Autodesk Fusion 360 part; units mm, degrees
(part 3 of 4)
sketch "Sketch4" plane through (0, 0, 0) normal (0, 0, -1) x (1, 0, 0) in component "Gear "
  line L0 (24.6001, -83.7803) -> (24.6516, -83.9556)
  line L1 (24.6516, -83.9556) -> (24.6577, -83.8757)
  line L2 (24.6577, -83.8757) -> (24.6976, -83.9421)
  line L3 (24.6976, -83.9421) -> (24.6684, -83.7391)
  spline S0 degree 5 poles (24.6684, -83.7391) (24.7188, -83.1041) (24.8375, -81.8379) (25.0626, -80.0652) (25.4578, -77.9934) (26.1207, -75.9415) (26.9802, -74.4769) (28.0438, -73.6781) (29.3213, -73.5772) (30.8056, -74.151) (32.4625, -75.3371) (33.9214, -76.7307) (35.082, -78.0047) (35.8789, -78.9461) (36.2729, -79.4266) knots 0.006357 0.006357 0.006357 0.006357 0.006357 0.006357 0.1 0.2 0.3 0.4 0.5 0.6 0.7 0.8 0.9 0.994293 0.994293 0.994293 0.994293 0.994293 0.994293
  line L4 (36.2729, -79.4266) -> (36.3488, -79.5928)
  line L5 (36.3488, -79.5928) -> (36.3435, -79.5128)
  line L6 (36.3435, -79.5128) -> (36.3924, -79.5729)
  line L7 (36.3924, -79.5729) -> (36.3346, -79.376)
  spline S1 degree 5 poles (36.3346, -79.376) (36.2942, -78.7403) (36.2315, -77.4702) (36.202, -75.6835) (36.2983, -73.5765) (36.6624, -71.4511) (37.3048, -69.8791) (38.2439, -68.9371) (39.494, -68.6554) (41.0448, -69.0122) (42.8537, -69.9504) (44.4961, -71.1222) (45.8261, -72.2181) (46.7489, -73.0365) (47.2073, -73.456) knots 0.006357 0.006357 0.006357 0.006357 0.006357 0.006357 0.1 0.2 0.3 0.4 0.5 0.6 0.7 0.8 0.9 0.994293 0.994293 0.994293 0.994293 0.994293 0.994293
  line L8 (47.2073, -73.456) -> (47.3061, -73.6097)
  line L9 (47.3061, -73.6097) -> (47.2894, -73.5313)
  line L10 (47.2894, -73.5313) -> (47.3464, -73.5838)
  line L11 (47.3464, -73.5838) -> (47.2612, -73.3971)
  spline S2 degree 5 poles (47.2612, -73.3971) (47.1307, -72.7737) (46.8878, -71.5254) (46.6044, -69.761) (46.3998, -67.6618) (46.4578, -65.5062) (46.8699, -63.8588) (47.6654, -62.7928) (48.8627, -62.336) (50.4485, -62.4685) (52.3725, -63.1396) (54.1649, -64.0658) (55.6374, -64.9613) (56.6673, -65.64) (57.1807, -65.99) knots 0.006357 0.006357 0.006357 0.006357 0.006357 0.006357 0.1 0.2 0.3 0.4 0.5 0.6 0.7 0.8 0.9 0.994293 0.994293 0.994293 0.994293 0.994293 0.994293
  line L12 (57.1807, -65.99) -> (57.3003, -66.1281)
  line L13 (57.3003, -66.1281) -> (57.2727, -66.0529)
  line L14 (57.2727, -66.0529) -> (57.3365, -66.0967)
  line L15 (57.3365, -66.0967) -> (57.2256, -65.9241)
  spline S3 degree 5 poles (57.2256, -65.9241) (57.0077, -65.3255) (56.5897, -64.1245) (56.0581, -62.4185) (55.5568, -60.3697) (55.3074, -58.2279) (55.4809, -56.5386) (56.1166, -55.3701) (57.2366, -54.7476) (58.8252, -54.6531) (60.8251, -55.0436) (62.7311, -55.7052) (64.316, -56.382) (65.432, -56.9073) (65.99, -57.1807) knots 0.006357 0.006357 0.006357 0.006357 0.006357 0.006357 0.1 0.2 0.3 0.4 0.5 0.6 0.7 0.8 0.9 0.994293 0.994293 0.994293 0.994293 0.994293 0.994293
  line L16 (65.99, -57.1807) -> (66.1281, -57.3003)
  line L17 (66.1281, -57.3003) -> (66.09, -57.2298)
  line L18 (66.09, -57.2298) -> (66.1595, -57.2641)
  line L19 (66.1595, -57.2641) -> (66.0251, -57.109)
  spline S4 degree 5 poles (66.0251, -57.109) (65.7243, -56.5476) (65.1396, -55.4182) (64.3705, -53.8052) (63.5828, -51.8487) (63.0312, -49.7641) (62.9624, -48.0673) (63.4254, -46.8203) (64.4455, -46.0448) (66.0044, -45.7251) (68.0395, -45.827) (70.0203, -46.2107) (71.6854, -46.655) (72.8648, -47.0161) (73.456, -47.2073) knots 0.006357 0.006357 0.006357 0.006357 0.006357 0.006357 0.1 0.2 0.3 0.4 0.5 0.6 0.7 0.8 0.9 0.994293 0.994293 0.994293 0.994293 0.994293 0.994293
  line L20 (73.456, -47.2073) -> (73.6097, -47.3061)
  line L21 (73.6097, -47.3061) -> (73.562, -47.2417)
  line L22 (73.562, -47.2417) -> (73.6356, -47.2657)
  line L23 (73.6356, -47.2657) -> (73.4805, -47.1314)
  spline S5 degree 5 poles (73.4805, -47.1314) (73.1028, -46.6185) (72.3634, -45.5838) (71.3726, -44.0967) (70.3145, -42.2722) (69.4718, -40.2873) (69.1623, -38.6176) (69.443, -37.3174) (70.3423, -36.4045) (71.8399, -35.8663) (73.8688, -35.6775) (75.884, -35.7754) (77.5954, -35.9782) (78.8142, -36.1678) (79.4266, -36.2729) knots 0.006357 0.006357 0.006357 0.006357 0.006357 0.006357 0.1 0.2 0.3 0.4 0.5 0.6 0.7 0.8 0.9 0.994293 0.994293 0.994293 0.994293 0.994293 0.994293
  line L24 (79.4266, -36.2729) -> (79.5928, -36.3488)
  line L25 (79.5928, -36.3488) -> (79.5364, -36.2919)
  line L26 (79.5364, -36.2919) -> (79.6127, -36.3052)
  line L27 (79.6127, -36.3052) -> (79.4401, -36.1943)
  spline S6 degree 5 poles (79.4401, -36.1943) (78.9933, -35.7403) (78.1141, -34.8215) (76.9218, -33.4905) (75.6147, -31.8351) (74.4981, -29.9904) (73.9542, -28.3817) (74.047, -27.0548) (74.8073, -26.0232) (76.213, -25.2773) (78.1944, -24.8018) (80.203, -24.6118) (81.9259, -24.569) (83.1592, -24.5832) (83.7803, -24.6001) knots 0.006357 0.006357 0.006357 0.006357 0.006357 0.006357 0.1 0.2 0.3 0.4 0.5 0.6 0.7 0.8 0.9 0.994293 0.994293 0.994293 0.994293 0.994293 0.994293
  line L28 (83.7803, -24.6001) -> (83.9556, -24.6516)
  line L29 (83.9556, -24.6516) -> (83.8917, -24.6033)
  line L30 (83.8917, -24.6033) -> (83.9691, -24.6056)
  line L31 (83.9691, -24.6056) -> (83.7825, -24.5204)
  spline S7 degree 5 poles (83.7825, -24.5204) (83.2756, -24.1346) (82.2746, -23.3503) (80.905, -22.2025) (79.3757, -20.75) (78.0079, -19.0829) (77.2405, -17.568) (77.1436, -16.2414) (77.7493, -15.1122) (79.0346, -14.1738) (80.9282, -13.4211) (82.8893, -12.9472) (84.5885, -12.6597) (85.8113, -12.4982) (86.4285, -12.4265) knots 0.006357 0.006357 0.006357 0.006357 0.006357 0.006357 0.1 0.2 0.3 0.4 0.5 0.6 0.7 0.8 0.9 0.994293 0.994293 0.994293 0.994293 0.994293 0.994293
  line L32 (86.4285, -12.4265) -> (86.6094, -12.4525)
  line L33 (86.6094, -12.4525) -> (86.5392, -12.4138)
  line L34 (86.5392, -12.4138) -> (86.6162, -12.4051)
  line L35 (86.6162, -12.4051) -> (86.4193, -12.3473)
  spline S8 degree 5 poles (86.4193, -12.3473) (85.8627, -12.0376) (84.7603, -11.4037) (83.2413, -10.4625) (81.5208, -9.2424) (79.9297, -7.787) (78.9545, -6.3967) (78.6698, -5.0974) (79.1086, -3.8935) (80.2473, -2.7817) (82.0144, -1.7672) (83.8882, -1.0191) (85.5292, -0.4926) (86.7166, -0.1588) (87.3173, 0) knots 0.006357 0.006357 0.006357 0.006357 0.006357 0.006357 0.1 0.2 0.3 0.4 0.5 0.6 0.7 0.8 0.9 0.994293 0.994293 0.994293 0.994293 0.994293 0.994293
  line L36 (87.3173, 0) -> (87.5, 0)
  line L37 (87.5, 0) -> (87.4251, 0.0284)
  line L38 (87.4251, 0.0284) -> (87.5, 0.0479)
  line L39 (87.5, 0.0479) -> (87.2969, 0.0771)
  spline S9 degree 5 poles (87.2969, 0.0771) (86.7019, 0.3044) (85.5204, 0.775) (83.883, 1.4905) (82.0064, 2.4533) (80.2243, 3.6674) (79.0612, 4.9048) (78.5945, 6.1503) (78.8575, 7.4045) (79.8263, 8.667) (81.4312, 9.9227) (83.1793, 10.9298) (84.7287, 11.6844) (85.8565, 12.1839) (86.4285, 12.4265) knots 0.006357 0.006357 0.006357 0.006357 0.006357 0.006357 0.1 0.2 0.3 0.4 0.5 0.6 0.7 0.8 0.9 0.994293 0.994293 0.994293 0.994293 0.994293 0.994293
  line L40 (86.4285, 12.4265) -> (86.6094, 12.4525)
  line L41 (86.6094, 12.4525) -> (86.5312, 12.47)
  line L42 (86.5312, 12.47) -> (86.6025, 12.5)
  line L43 (86.6025, 12.5) -> (86.3974, 12.5)
  spline S10 degree 5 poles (86.3974, 12.5) (85.776, 12.6403) (84.5397, 12.938) (82.817, 13.4131) (80.8225, 14.099) (78.8858, 15.0472) (77.5585, 16.1064) (76.9192, 17.2729) (77.0011, 18.5517) (77.7804, 19.9392) (79.1902, 21.4105) (80.7772, 22.6562) (82.2035, 23.6237) (83.2487, 24.2785) (83.7803, 24.6001) knots 0.006357 0.006357 0.006357 0.006357 0.006357 0.006357 0.1 0.2 0.3 0.4 0.5 0.6 0.7 0.8 0.9 0.994293 0.994293 0.994293 0.994293 0.994293 0.994293
  line L44 (83.7803, 24.6001) -> (83.9556, 24.6516)
  line L45 (83.9556, 24.6516) -> (83.8757, 24.6577)
  line L46 (83.8757, 24.6577) -> (83.9421, 24.6976)
  line L47 (83.9421, 24.6976) -> (83.7391, 24.6684)
  spline S11 degree 5 poles (83.7391, 24.6684) (83.1041, 24.7188) (81.8379, 24.8375) (80.0652, 25.0626) (77.9934, 25.4578) (75.9415, 26.1207) (74.4769, 26.9802) (73.6781, 28.0438) (73.5772, 29.3213) (74.151, 30.8056) (75.3371, 32.4625) (76.7307, 33.9214) (78.0047, 35.082) (78.9461, 35.8789) (79.4266, 36.2729) knots 0.006357 0.006357 0.006357 0.006357 0.006357 0.006357 0.1 0.2 0.3 0.4 0.5 0.6 0.7 0.8 0.9 0.994293 0.994293 0.994293 0.994293 0.994293 0.994293
  line L48 (79.4266, 36.2729) -> (79.5928, 36.3488)
  line L49 (79.5928, 36.3488) -> (79.5128, 36.3435)
  line L50 (79.5128, 36.3435) -> (79.5729, 36.3924)
  line L51 (79.5729, 36.3924) -> (79.376, 36.3346)
  spline S12 degree 5 poles (79.376, 36.3346) (78.7403, 36.2942) (77.4702, 36.2315) (75.6835, 36.202) (73.5765, 36.2983) (71.4511, 36.6624) (69.8791, 37.3048) (68.9371, 38.2439) (68.6554, 39.494) (69.0122, 41.0448) (69.9504, 42.8537) (71.1222, 44.4961) (72.2181, 45.8261) (73.0365, 46.7489) (73.456, 47.2073) knots 0.006357 0.006357 0.006357 0.006357 0.006357 0.006357 0.1 0.2 0.3 0.4 0.5 0.6 0.7 0.8 0.9 0.994293 0.994293 0.994293 0.994293 0.994293 0.994293
  line L52 (73.456, 47.2073) -> (73.6097, 47.3061)
  line L53 (73.6097, 47.3061) -> (73.5313, 47.2894)
  line L54 (73.5313, 47.2894) -> (73.5838, 47.3464)
  line L55 (73.5838, 47.3464) -> (73.3971, 47.2612)
  spline S13 degree 5 poles (73.3971, 47.2612) (72.7737, 47.1307) (71.5254, 46.8878) (69.761, 46.6044) (67.6618, 46.3998) (65.5062, 46.4578) (63.8588, 46.8699) (62.7928, 47.6654) (62.336, 48.8627) (62.4685, 50.4485) (63.1396, 52.3725) (64.0658, 54.1649) (64.9613, 55.6374) (65.64, 56.6673) (65.99, 57.1807) knots 0.006357 0.006357 0.006357 0.006357 0.006357 0.006357 0.1 0.2 0.3 0.4 0.5 0.6 0.7 0.8 0.9 0.994293 0.994293 0.994293 0.994293 0.994293 0.994293
  line L56 (65.99, 57.1807) -> (66.1281, 57.3003)
  line L57 (66.1281, 57.3003) -> (66.0529, 57.2727)
  line L58 (66.0529, 57.2727) -> (66.0967, 57.3365)
  line L59 (66.0967, 57.3365) -> (65.9241, 57.2256)
  spline S14 degree 5 poles (65.9241, 57.2256) (65.3255, 57.0077) (64.1245, 56.5897) (62.4185, 56.0581) (60.3697, 55.5568) (58.2279, 55.3074) (56.5386, 55.4809) (55.3701, 56.1166) (54.7476, 57.2366) (54.6531, 58.8252) (55.0436, 60.8251) (55.7052, 62.7311) (56.382, 64.316) (56.9073, 65.432) (57.1807, 65.99) knots 0.006357 0.006357 0.006357 0.006357 0.006357 0.006357 0.1 0.2 0.3 0.4 0.5 0.6 0.7 0.8 0.9 0.994293 0.994293 0.994293 0.994293 0.994293 0.994293
  line L60 (57.1807, 65.99) -> (57.3003, 66.1281)
  line L61 (57.3003, 66.1281) -> (57.2298, 66.09)
  line L62 (57.2298, 66.09) -> (57.2641, 66.1595)
  line L63 (57.2641, 66.1595) -> (57.109, 66.0251)
  spline S15 degree 5 poles (57.109, 66.0251) (56.5476, 65.7243) (55.4182, 65.1396) (53.8052, 64.3705) (51.8487, 63.5828) (49.7641, 63.0312) (48.0673, 62.9624) (46.8203, 63.4254) (46.0448, 64.4455) (45.7251, 66.0044) (45.827, 68.0395) (46.2107, 70.0203) (46.655, 71.6854) (47.0161, 72.8648) (47.2073, 73.456) knots 0.006357 0.006357 0.006357 0.006357 0.006357 0.006357 0.1 0.2 0.3 0.4 0.5 0.6 0.7 0.8 0.9 0.994293 0.994293 0.994293 0.994293 0.994293 0.994293
  line L64 (47.2073, 73.456) -> (47.3061, 73.6097)
  line L65 (47.3061, 73.6097) -> (47.2417, 73.562)
  line L66 (47.2417, 73.562) -> (47.2657, 73.6356)
  line L67 (47.2657, 73.6356) -> (47.1314, 73.4805)
  spline S16 degree 5 poles (47.1314, 73.4805) (46.6185, 73.1028) (45.5838, 72.3634) (44.0967, 71.3726) (42.2722, 70.3145) (40.2873, 69.4718) (38.6176, 69.1623) (37.3174, 69.443) (36.4045, 70.3423) (35.8663, 71.8399) (35.6775, 73.8688) (35.7754, 75.884) (35.9782, 77.5954) (36.1678, 78.8142) (36.2729, 79.4266) knots 0.006357 0.006357 0.006357 0.006357 0.006357 0.006357 0.1 0.2 0.3 0.4 0.5 0.6 0.7 0.8 0.9 0.994293 0.994293 0.994293 0.994293 0.994293 0.994293
  line L68 (36.2729, 79.4266) -> (36.3488, 79.5928)
  line L69 (36.3488, 79.5928) -> (36.2919, 79.5364)
  line L70 (36.2919, 79.5364) -> (36.3052, 79.6127)
  line L71 (36.3052, 79.6127) -> (36.1943, 79.4401)
  spline S17 degree 5 poles (36.1943, 79.4401) (35.7403, 78.9933) (34.8215, 78.1141) (33.4905, 76.9218) (31.8351, 75.6147) (29.9904, 74.4981) (28.3817, 73.9542) (27.0548, 74.047) (26.0232, 74.8073) (25.2773, 76.213) (24.8018, 78.1944) (24.6118, 80.203) (24.569, 81.9259) (24.5832, 83.1592) (24.6001, 83.7803) knots 0.006357 0.006357 0.006357 0.006357 0.006357 0.006357 0.1 0.2 0.3 0.4 0.5 0.6 0.7 0.8 0.9 0.994293 0.994293 0.994293 0.994293 0.994293 0.994293
  line L72 (24.6001, 83.7803) -> (24.6516, 83.9556)
  line L73 (24.6516, 83.9556) -> (24.6033, 83.8917)
  line L74 (24.6033, 83.8917) -> (24.6056, 83.9691)
  line L75 (24.6056, 83.9691) -> (24.5204, 83.7825)
  spline S18 degree 5 poles (24.5204, 83.7825) (24.1346, 83.2756) (23.3503, 82.2746) (22.2025, 80.905) (20.75, 79.3757) (19.0829, 78.0079) (17.568, 77.2405) (16.2414, 77.1436) (15.1122, 77.7493) (14.1738, 79.0346) (13.4211, 80.9282) (12.9472, 82.8893) (12.6597, 84.5885) (12.4982, 85.8113) (12.4265, 86.4285) knots 0.006357 0.006357 0.006357 0.006357 0.006357 0.006357 0.1 0.2 0.3 0.4 0.5 0.6 0.7 0.8 0.9 0.994293 0.994293 0.994293 0.994293 0.994293 0.994293
  line L76 (12.4265, 86.4285) -> (12.4525, 86.6094)
  line L77 (12.4525, 86.6094) -> (12.4138, 86.5392)
  line L78 (12.4138, 86.5392) -> (12.4051, 86.6162)
  line L79 (12.4051, 86.6162) -> (12.3473, 86.4193)
  spline S19 degree 5 poles (12.3473, 86.4193) (12.0376, 85.8627) (11.4037, 84.7603) (10.4625, 83.2413) (9.2424, 81.5208) (7.787, 79.9297) (6.3967, 78.9545) (5.0974, 78.6698) (3.8935, 79.1086) (2.7817, 80.2473) (1.7672, 82.0144) (1.0191, 83.8882) (0.4926, 85.5292) (0.1588, 86.7166) (0, 87.3173) knots 0.006357 0.006357 0.006357 0.006357 0.006357 0.006357 0.1 0.2 0.3 0.4 0.5 0.6 0.7 0.8 0.9 0.994293 0.994293 0.994293 0.994293 0.994293 0.994293
  line L80 (0, 87.3173) -> (0, 87.5)
  line L81 (0, 87.5) -> (-0.0284, 87.4251)
  line L82 (-0.0284, 87.4251) -> (-0.0479, 87.5)
  line L83 (-0.0479, 87.5) -> (-0.0771, 87.2969)
  spline S20 degree 5 poles (-0.0771, 87.2969) (-0.3044, 86.7019) (-0.775, 85.5204) (-1.4905, 83.883) (-2.4533, 82.0064) (-3.6674, 80.2243) (-4.9048, 79.0612) (-6.1503, 78.5945) (-7.4045, 78.8575) (-8.667, 79.8263) (-9.9227, 81.4312) (-10.9298, 83.1793) (-11.6844, 84.7287) (-12.1839, 85.8565) (-12.4265, 86.4285) knots 0.006357 0.006357 0.006357 0.006357 0.006357 0.006357 0.1 0.2 0.3 0.4 0.5 0.6 0.7 0.8 0.9 0.994293 0.994293 0.994293 0.994293 0.994293 0.994293
  line L84 (-12.4265, 86.4285) -> (-12.4525, 86.6094)
  line L85 (-12.4525, 86.6094) -> (-12.47, 86.5312)
  line L86 (-12.47, 86.5312) -> (-12.5, 86.6025)
  line L87 (-12.5, 86.6025) -> (-12.5, 86.3974)
  spline S21 degree 5 poles (-12.5, 86.3974) (-12.6403, 85.776) (-12.938, 84.5397) (-13.4131, 82.817) (-14.099, 80.8225) (-15.0472, 78.8858) (-16.1064, 77.5585) (-17.2729, 76.9192) (-18.5517, 77.0011) (-19.9392, 77.7804) (-21.4105, 79.1902) (-22.6562, 80.7772) (-23.6237, 82.2035) (-24.2785, 83.2487) (-24.6001, 83.7803) knots 0.006357 0.006357 0.006357 0.006357 0.006357 0.006357 0.1 0.2 0.3 0.4 0.5 0.6 0.7 0.8 0.9 0.994293 0.994293 0.994293 0.994293 0.994293 0.994293
  line L88 (-24.6001, 83.7803) -> (-24.6516, 83.9556)
  line L89 (-24.6516, 83.9556) -> (-24.6577, 83.8757)
  line L90 (-24.6577, 83.8757) -> (-24.6976, 83.9421)
  line L91 (-24.6976, 83.9421) -> (-24.6684, 83.7391)
  spline S22 degree 5 poles (-24.6684, 83.7391) (-24.7188, 83.1041) (-24.8375, 81.8379) (-25.0626, 80.0652) (-25.4578, 77.9934) (-26.1207, 75.9415) (-26.9802, 74.4769) (-28.0438, 73.6781) (-29.3213, 73.5772) (-30.8056, 74.151) (-32.4625, 75.3371) (-33.9214, 76.7307) (-35.082, 78.0047) (-35.8789, 78.9461) (-36.2729, 79.4266) knots 0.006357 0.006357 0.006357 0.006357 0.006357 0.006357 0.1 0.2 0.3 0.4 0.5 0.6 0.7 0.8 0.9 0.994293 0.994293 0.994293 0.994293 0.994293 0.994293
  line L92 (-36.2729, 79.4266) -> (-36.3488, 79.5928)
  line L93 (-36.3488, 79.5928) -> (-36.3435, 79.5128)
  line L94 (-36.3435, 79.5128) -> (-36.3924, 79.5729)
  line L95 (-36.3924, 79.5729) -> (-36.3346, 79.376)
  spline S23 degree 5 poles (-36.3346, 79.376) (-36.2942, 78.7403) (-36.2315, 77.4702) (-36.202, 75.6835) (-36.2983, 73.5765) (-36.6624, 71.4511) (-37.3048, 69.8791) (-38.2439, 68.9371) (-39.494, 68.6554) (-41.0448, 69.0122) (-42.8537, 69.9504) (-44.4961, 71.1222) (-45.8261, 72.2181) (-46.7489, 73.0365) (-47.2073, 73.456) knots 0.006357 0.006357 0.006357 0.006357 0.006357 0.006357 0.1 0.2 0.3 0.4 0.5 0.6 0.7 0.8 0.9 0.994293 0.994293 0.994293 0.994293 0.994293 0.994293
  line L96 (-47.2073, 73.456) -> (-47.3061, 73.6097)
  line L97 (-47.3061, 73.6097) -> (-47.2894, 73.5313)
  line L98 (-47.2894, 73.5313) -> (-47.3464, 73.5838)
  line L99 (-47.3464, 73.5838) -> (-47.2612, 73.3971)
  spline S24 degree 5 poles (-47.2612, 73.3971) (-47.1307, 72.7737) (-46.8878, 71.5254) (-46.6044, 69.761) (-46.3998, 67.6618) (-46.4578, 65.5062) (-46.8699, 63.8588) (-47.6654, 62.7928) (-48.8627, 62.336) (-50.4485, 62.4685) (-52.3725, 63.1396) (-54.1649, 64.0658) (-55.6374, 64.9613) (-56.6673, 65.64) (-57.1807, 65.99) knots 0.006357 0.006357 0.006357 0.006357 0.006357 0.006357 0.1 0.2 0.3 0.4 0.5 0.6 0.7 0.8 0.9 0.994293 0.994293 0.994293 0.994293 0.994293 0.994293
  line L100 (-57.1807, 65.99) -> (-57.3003, 66.1281)
  line L101 (-57.3003, 66.1281) -> (-57.2727, 66.0529)
  line L102 (-57.2727, 66.0529) -> (-57.3365, 66.0967)
  line L103 (-57.3365, 66.0967) -> (-57.2256, 65.9241)
  spline S25 degree 5 poles (-57.2256, 65.9241) (-57.0077, 65.3255) (-56.5897, 64.1245) (-56.0581, 62.4185) (-55.5568, 60.3697) (-55.3074, 58.2279) (-55.4809, 56.5386) (-56.1166, 55.3701) (-57.2366, 54.7476) (-58.8252, 54.6531) (-60.8251, 55.0436) (-62.7311, 55.7052) (-64.316, 56.382) (-65.432, 56.9073) (-65.99, 57.1807) knots 0.006357 0.006357 0.006357 0.006357 0.006357 0.006357 0.1 0.2 0.3 0.4 0.5 0.6 0.7 0.8 0.9 0.994293 0.994293 0.994293 0.994293 0.994293 0.994293
  line L104 (-65.99, 57.1807) -> (-66.1281, 57.3003)
  line L105 (-66.1281, 57.3003) -> (-66.09, 57.2298)
  line L106 (-66.09, 57.2298) -> (-66.1595, 57.2641)
  line L107 (-66.1595, 57.2641) -> (-66.0251, 57.109)
  spline S26 degree 5 poles (-66.0251, 57.109) (-65.7243, 56.5476) (-65.1396, 55.4182) (-64.3705, 53.8052) (-63.5828, 51.8487) (-63.0312, 49.7641) (-62.9624, 48.0673) (-63.4254, 46.8203) (-64.4455, 46.0448) (-66.0044, 45.7251) (-68.0395, 45.827) (-70.0203, 46.2107) (-71.6854, 46.655) (-72.8648, 47.0161) (-73.456, 47.2073) knots 0.006357 0.006357 0.006357 0.006357 0.006357 0.006357 0.1 0.2 0.3 0.4 0.5 0.6 0.7 0.8 0.9 0.994293 0.994293 0.994293 0.994293 0.994293 0.994293
  line L108 (-73.456, 47.2073) -> (-73.6097, 47.3061)
  line L109 (-73.6097, 47.3061) -> (-73.562, 47.2417)
  line L110 (-73.562, 47.2417) -> (-73.6356, 47.2657)
  line L111 (-73.6356, 47.2657) -> (-73.4805, 47.1314)
  spline S27 degree 5 poles (-73.4805, 47.1314) (-73.1028, 46.6185) (-72.3634, 45.5838) (-71.3726, 44.0967) (-70.3145, 42.2722) (-69.4718, 40.2873) (-69.1623, 38.6176) (-69.443, 37.3174) (-70.3423, 36.4045) (-71.8399, 35.8663) (-73.8688, 35.6775) (-75.884, 35.7754) (-77.5954, 35.9782) (-78.8142, 36.1678) (-79.4266, 36.2729) knots 0.006357 0.006357 0.006357 0.006357 0.006357 0.006357 0.1 0.2 0.3 0.4 0.5 0.6 0.7 0.8 0.9 0.994293 0.994293 0.994293 0.994293 0.994293 0.994293
  line L112 (-79.4266, 36.2729) -> (-79.5928, 36.3488)
  line L113 (-79.5928, 36.3488) -> (-79.5364, 36.2919)
  line L114 (-79.5364, 36.2919) -> (-79.6127, 36.3052)
  line L115 (-79.6127, 36.3052) -> (-79.4401, 36.1943)
  spline S28 degree 5 poles (-79.4401, 36.1943) (-78.9933, 35.7403) (-78.1141, 34.8215) (-76.9218, 33.4905) (-75.6147, 31.8351) (-74.4981, 29.9904) (-73.9542, 28.3817) (-74.047, 27.0548) (-74.8073, 26.0232) (-76.213, 25.2773) (-78.1944, 24.8018) (-80.203, 24.6118) (-81.9259, 24.569) (-83.1592, 24.5832) (-83.7803, 24.6001) knots 0.006357 0.006357 0.006357 0.006357 0.006357 0.006357 0.1 0.2 0.3 0.4 0.5 0.6 0.7 0.8 0.9 0.994293 0.994293 0.994293 0.994293 0.994293 0.994293
  line L116 (-83.7803, 24.6001) -> (-83.9556, 24.6516)
  line L117 (-83.9556, 24.6516) -> (-83.8917, 24.6033)
  line L118 (-83.8917, 24.6033) -> (-83.9691, 24.6056)
  line L119 (-83.9691, 24.6056) -> (-83.7825, 24.5204)
  spline S29 degree 5 poles (-83.7825, 24.5204) (-83.2756, 24.1346) (-82.2746, 23.3503) (-80.905, 22.2025) (-79.3757, 20.75) (-78.0079, 19.0829) (-77.2405, 17.568) (-77.1436, 16.2414) (-77.7493, 15.1122) (-79.0346, 14.1738) (-80.9282, 13.4211) (-82.8893, 12.9472) (-84.5885, 12.6597) (-85.8113, 12.4982) (-86.4285, 12.4265) knots 0.006357 0.006357 0.006357 0.006357 0.006357 0.006357 0.1 0.2 0.3 0.4 0.5 0.6 0.7 0.8 0.9 0.994293 0.994293 0.994293 0.994293 0.994293 0.994293
  line L120 (-86.4285, 12.4265) -> (-86.6094, 12.4525)
  line L121 (-86.6094, 12.4525) -> (-86.5392, 12.4138)
  line L122 (-86.5392, 12.4138) -> (-86.6162, 12.4051)
  line L123 (-86.6162, 12.4051) -> (-86.4193, 12.3473)
  spline S30 degree 5 poles (-86.4193, 12.3473) (-85.8627, 12.0376) (-84.7603, 11.4037) (-83.2413, 10.4625) (-81.5208, 9.2424) (-79.9297, 7.787) (-78.9545, 6.3967) (-78.6698, 5.0974) (-79.1086, 3.8935) (-80.2473, 2.7817) (-82.0144, 1.7672) (-83.8882, 1.0191) (-85.5292, 0.4926) (-86.7166, 0.1588) (-87.3173, 0) knots 0.006357 0.006357 0.006357 0.006357 0.006357 0.006357 0.1 0.2 0.3 0.4 0.5 0.6 0.7 0.8 0.9 0.994293 0.994293 0.994293 0.994293 0.994293 0.994293
  line L124 (-87.3173, 0) -> (-87.5, 0)
  line L125 (-87.5, 0) -> (-87.4251, -0.0284)
  line L126 (-87.4251, -0.0284) -> (-87.5, -0.0479)
  line L127 (-87.5, -0.0479) -> (-87.2969, -0.0771)
  spline S31 degree 5 poles (-87.2969, -0.0771) (-86.7019, -0.3044) (-85.5204, -0.775) (-83.883, -1.4905) (-82.0064, -2.4533) (-80.2243, -3.6674) (-79.0612, -4.9048) (-78.5945, -6.1503) (-78.8575, -7.4045) (-79.8263, -8.667) (-81.4312, -9.9227) (-83.1793, -10.9298) (-84.7287, -11.6844) (-85.8565, -12.1839) (-86.4285, -12.4265) knots 0.006357 0.006357 0.006357 0.006357 0.006357 0.006357 0.1 0.2 0.3 0.4 0.5 0.6 0.7 0.8 0.9 0.994293 0.994293 0.994293 0.994293 0.994293 0.994293
  line L128 (-86.4285, -12.4265) -> (-86.6094, -12.4525)
  line L129 (-86.6094, -12.4525) -> (-86.5312, -12.47)
  line L130 (-86.5312, -12.47) -> (-86.6025, -12.5)
  line L131 (-86.6025, -12.5) -> (-86.3974, -12.5)
  spline S32 degree 5 poles (-86.3974, -12.5) (-85.776, -12.6403) (-84.5397, -12.938) (-82.817, -13.4131) (-80.8225, -14.099) (-78.8858, -15.0472) (-77.5585, -16.1064) (-76.9192, -17.2729) (-77.0011, -18.5517) (-77.7804, -19.9392) (-79.1902, -21.4105) (-80.7772, -22.6562) (-82.2035, -23.6237) (-83.2487, -24.2785) (-83.7803, -24.6001) knots 0.006357 0.006357 0.006357 0.006357 0.006357 0.006357 0.1 0.2 0.3 0.4 0.5 0.6 0.7 0.8 0.9 0.994293 0.994293 0.994293 0.994293 0.994293 0.994293
  line L132 (-83.7803, -24.6001) -> (-83.9556, -24.6516)
  line L133 (-83.9556, -24.6516) -> (-83.8757, -24.6577)
  line L134 (-83.8757, -24.6577) -> (-83.9421, -24.6976)
  line L135 (-83.9421, -24.6976) -> (-83.7391, -24.6684)
  spline S33 degree 5 poles (-83.7391, -24.6684) (-83.1041, -24.7188) (-81.8379, -24.8375) (-80.0652, -25.0626) (-77.9934, -25.4578) (-75.9415, -26.1207) (-74.4769, -26.9802) (-73.6781, -28.0438) (-73.5772, -29.3213) (-74.151, -30.8056) (-75.3371, -32.4625) (-76.7307, -33.9214) (-78.0047, -35.082) (-78.9461, -35.8789) (-79.4266, -36.2729) knots 0.006357 0.006357 0.006357 0.006357 0.006357 0.006357 0.1 0.2 0.3 0.4 0.5 0.6 0.7 0.8 0.9 0.994293 0.994293 0.994293 0.994293 0.994293 0.994293
  line L136 (-79.4266, -36.2729) -> (-79.5928, -36.3488)
  line L137 (-79.5928, -36.3488) -> (-79.5128, -36.3435)
  line L138 (-79.5128, -36.3435) -> (-79.5729, -36.3924)
  line L139 (-79.5729, -36.3924) -> (-79.376, -36.3346)
  spline S34 degree 5 poles (-79.376, -36.3346) (-78.7403, -36.2942) (-77.4702, -36.2315) (-75.6835, -36.202) (-73.5765, -36.2983) (-71.4511, -36.6624) (-69.8791, -37.3048) (-68.9371, -38.2439) (-68.6554, -39.494) (-69.0122, -41.0448) (-69.9504, -42.8537) (-71.1222, -44.4961) (-72.2181, -45.8261) (-73.0365, -46.7489) (-73.456, -47.2073) knots 0.006357 0.006357 0.006357 0.006357 0.006357 0.006357 0.1 0.2 0.3 0.4 0.5 0.6 0.7 0.8 0.9 0.994293 0.994293 0.994293 0.994293 0.994293 0.994293
  line L140 (-73.456, -47.2073) -> (-73.6097, -47.3061)
  line L141 (-73.6097, -47.3061) -> (-73.5313, -47.2894)
  line L142 (-73.5313, -47.2894) -> (-73.5838, -47.3464)
  line L143 (-73.5838, -47.3464) -> (-73.3971, -47.2612)
  spline S35 degree 5 poles (-73.3971, -47.2612) (-72.7737, -47.1307) (-71.5254, -46.8878) (-69.761, -46.6044) (-67.6618, -46.3998) (-65.5062, -46.4578) (-63.8588, -46.8699) (-62.7928, -47.6654) (-62.336, -48.8627) (-62.4685, -50.4485) (-63.1396, -52.3725) (-64.0658, -54.1649) (-64.9613, -55.6374) (-65.64, -56.6673) (-65.99, -57.1807) knots 0.006357 0.006357 0.006357 0.006357 0.006357 0.006357 0.1 0.2 0.3 0.4 0.5 0.6 0.7 0.8 0.9 0.994293 0.994293 0.994293 0.994293 0.994293 0.994293
  line L144 (-65.99, -57.1807) -> (-66.1281, -57.3003)
  line L145 (-66.1281, -57.3003) -> (-66.0529, -57.2727)
  line L146 (-66.0529, -57.2727) -> (-66.0967, -57.3365)
  line L147 (-66.0967, -57.3365) -> (-65.9241, -57.2256)
  spline S36 degree 5 poles (-65.9241, -57.2256) (-65.3255, -57.0077) (-64.1245, -56.5897) (-62.4185, -56.0581) (-60.3697, -55.5568) (-58.2279, -55.3074) (-56.5386, -55.4809) (-55.3701, -56.1166) (-54.7476, -57.2366) (-54.6531, -58.8252) (-55.0436, -60.8251) (-55.7052, -62.7311) (-56.382, -64.316) (-56.9073, -65.432) (-57.1807, -65.99) knots 0.006357 0.006357 0.006357 0.006357 0.006357 0.006357 0.1 0.2 0.3 0.4 0.5 0.6 0.7 0.8 0.9 0.994293 0.994293 0.994293 0.994293 0.994293 0.994293
  line L148 (-57.1807, -65.99) -> (-57.3003, -66.1281)
  line L149 (-57.3003, -66.1281) -> (-57.2298, -66.09)
  line L150 (-57.2298, -66.09) -> (-57.2641, -66.1595)
  line L151 (-57.2641, -66.1595) -> (-57.109, -66.0251)
  spline S37 degree 5 poles (-57.109, -66.0251) (-56.5476, -65.7243) (-55.4182, -65.1396) (-53.8052, -64.3705) (-51.8487, -63.5828) (-49.7641, -63.0312) (-48.0673, -62.9624) (-46.8203, -63.4254) (-46.0448, -64.4455) (-45.7251, -66.0044) (-45.827, -68.0395) (-46.2107, -70.0203) (-46.655, -71.6854) (-47.0161, -72.8648) (-47.2073, -73.456) knots 0.006357 0.006357 0.006357 0.006357 0.006357 0.006357 0.1 0.2 0.3 0.4 0.5 0.6 0.7 0.8 0.9 0.994293 0.994293 0.994293 0.994293 0.994293 0.994293
  line L152 (-47.2073, -73.456) -> (-47.3061, -73.6097)
  line L153 (-47.3061, -73.6097) -> (-47.2417, -73.562)
  line L154 (-47.2417, -73.562) -> (-47.2657, -73.6356)
  line L155 (-47.2657, -73.6356) -> (-47.1314, -73.4805)
  spline S38 degree 5 poles (-47.1314, -73.4805) (-46.6185, -73.1028) (-45.5838, -72.3634) (-44.0967, -71.3726) (-42.2722, -70.3145) (-40.2873, -69.4718) (-38.6176, -69.1623) (-37.3174, -69.443) (-36.4045, -70.3423) (-35.8663, -71.8399) (-35.6775, -73.8688) (-35.7754, -75.884) (-35.9782, -77.5954) (-36.1678, -78.8142) (-36.2729, -79.4266) knots 0.006357 0.006357 0.006357 0.006357 0.006357 0.006357 0.1 0.2 0.3 0.4 0.5 0.6 0.7 0.8 0.9 0.994293 0.994293 0.994293 0.994293 0.994293 0.994293
  line L156 (-36.2729, -79.4266) -> (-36.3488, -79.5928)
  line L157 (-36.3488, -79.5928) -> (-36.2919, -79.5364)
  line L158 (-36.2919, -79.5364) -> (-36.3052, -79.6127)
  line L159 (-36.3052, -79.6127) -> (-36.1943, -79.4401)
  spline S39 degree 5 poles (-36.1943, -79.4401) (-35.7403, -78.9933) (-34.8215, -78.1141) (-33.4905, -76.9218) (-31.8351, -75.6147) (-29.9904, -74.4981) (-28.3817, -73.9542) (-27.0548, -74.047) (-26.0232, -74.8073) (-25.2773, -76.213) (-24.8018, -78.1944) (-24.6118, -80.203) (-24.569, -81.9259) (-24.5832, -83.1592) (-24.6001, -83.7803) knots 0.006357 0.006357 0.006357 0.006357 0.006357 0.006357 0.1 0.2 0.3 0.4 0.5 0.6 0.7 0.8 0.9 0.994293 0.994293 0.994293 0.994293 0.994293 0.994293
  line L160 (-24.6001, -83.7803) -> (-24.6516, -83.9556)
  line L161 (-24.6516, -83.9556) -> (-24.6033, -83.8917)
  line L162 (-24.6033, -83.8917) -> (-24.6056, -83.9691)
  line L163 (-24.6056, -83.9691) -> (-24.5204, -83.7825)
  spline S40 degree 5 poles (-24.5204, -83.7825) (-24.1346, -83.2756) (-23.3503, -82.2746) (-22.2025, -80.905) (-20.75, -79.3757) (-19.0829, -78.0079) (-17.568, -77.2405) (-16.2414, -77.1436) (-15.1122, -77.7493) (-14.1738, -79.0346) (-13.4211, -80.9282) (-12.9472, -82.8893) (-12.6597, -84.5885) (-12.4982, -85.8113) (-12.4265, -86.4285) knots 0.006357 0.006357 0.006357 0.006357 0.006357 0.006357 0.1 0.2 0.3 0.4 0.5 0.6 0.7 0.8 0.9 0.994293 0.994293 0.994293 0.994293 0.994293 0.994293
  line L164 (-12.4265, -86.4285) -> (-12.4525, -86.6094)
  line L165 (-12.4525, -86.6094) -> (-12.4138, -86.5392)
  line L166 (-12.4138, -86.5392) -> (-12.4051, -86.6162)
  line L167 (-12.4051, -86.6162) -> (-12.3473, -86.4193)
  spline S41 degree 5 poles (-12.3473, -86.4193) (-12.0376, -85.8627) (-11.4037, -84.7603) (-10.4625, -83.2413) (-9.2424, -81.5208) (-7.787, -79.9297) (-6.3967, -78.9545) (-5.0974, -78.6698) (-3.8935, -79.1086) (-2.7817, -80.2473) (-1.7672, -82.0144) (-1.0191, -83.8882) (-0.4926, -85.5292) (-0.1588, -86.7166) (0, -87.3173) knots 0.006357 0.006357 0.006357 0.006357 0.006357 0.006357 0.1 0.2 0.3 0.4 0.5 0.6 0.7 0.8 0.9 0.994293 0.994293 0.994293 0.994293 0.994293 0.994293
  line L168 (0, -87.3173) -> (0, -87.5)
  line L169 (0, -87.5) -> (0.0284, -87.4251)
  line L170 (0.0284, -87.4251) -> (0.0479, -87.5)
  line L171 (0.0479, -87.5) -> (0.0771, -87.2969)
  spline S42 degree 5 poles (0.0771, -87.2969) (0.3044, -86.7019) (0.775, -85.5204) (1.4905, -83.883) (2.4533, -82.0064) (3.6674, -80.2243) (4.9048, -79.0612) (6.1503, -78.5945) (7.4045, -78.8575) (8.667, -79.8263) (9.9227, -81.4312) (10.9298, -83.1793) (11.6844, -84.7287) (12.1839, -85.8565) (12.4265, -86.4285) knots 0.006357 0.006357 0.006357 0.006357 0.006357 0.006357 0.1 0.2 0.3 0.4 0.5 0.6 0.7 0.8 0.9 0.994293 0.994293 0.994293 0.994293 0.994293 0.994293
  line L172 (12.4265, -86.4285) -> (12.4525, -86.6094)
  line L173 (12.4525, -86.6094) -> (12.47, -86.5312)
  line L174 (12.47, -86.5312) -> (12.5, -86.6025)
  line L175 (12.5, -86.6025) -> (12.5, -86.3974)
  spline S43 degree 5 poles (12.5, -86.3974) (12.6403, -85.776) (12.938, -84.5397) (13.4131, -82.817) (14.099, -80.8225) (15.0472, -78.8858) (16.1064, -77.5585) (17.2729, -76.9192) (18.5517, -77.0011) (19.9392, -77.7804) (21.4105, -79.1902) (22.6562, -80.7772) (23.6237, -82.2035) (24.2785, -83.2487) (24.6001, -83.7803) knots 0.006357 0.006357 0.006357 0.006357 0.006357 0.006357 0.1 0.2 0.3 0.4 0.5 0.6 0.7 0.8 0.9 0.994293 0.994293 0.994293 0.994293 0.994293 0.994293
  circle A0 centre (0, 0) radius 17.5
  dimension "d18" = 35
  constraint coincident A0.centre origin
  measures "d18" diameter of A0
extrude "Extrude4" add sketch "Sketch4" along normal blind 130 separate body contours A0 makes body 4 in component "Gear "
sketch "Sketch5" plane through (0, 0, 2) normal (0, 0, 1) x (-1, 0, 0) in component "Gear "
  line L0 (-24.6516, -83.9556) -> (-24.6001, -83.7803)
  spline S0 degree 5 poles (-24.6001, -83.7803) (-24.2785, -83.2487) (-23.6237, -82.2035) (-22.6562, -80.7772) (-21.4105, -79.1902) (-19.9392, -77.7804) (-18.5517, -77.0011) (-17.2729, -76.9192) (-16.1064, -77.5585) (-15.0472, -78.8858) (-14.099, -80.8225) (-13.4131, -82.817) (-12.938, -84.5397) (-12.6403, -85.776) (-12.5, -86.3974) knots -0.994293 -0.994293 -0.994293 -0.994293 -0.994293 -0.994293 -0.9 -0.8 -0.7 -0.6 -0.5 -0.4 -0.3 -0.2 -0.1 -0.006357 -0.006357 -0.006357 -0.006357 -0.006357 -0.006357
  line L1 (-12.5, -86.3974) -> (-12.5, -86.6025)
  line L2 (-12.5, -86.6025) -> (-12.47, -86.5312)
  line L3 (-12.47, -86.5312) -> (-12.4525, -86.6094)
  line L4 (-12.4525, -86.6094) -> (-12.4265, -86.4285)
  spline S1 degree 5 poles (-12.4265, -86.4285) (-12.1839, -85.8565) (-11.6844, -84.7287) (-10.9298, -83.1793) (-9.9227, -81.4312) (-8.667, -79.8263) (-7.4045, -78.8575) (-6.1503, -78.5945) (-4.9048, -79.0612) (-3.6674, -80.2243) (-2.4533, -82.0064) (-1.4905, -83.883) (-0.775, -85.5204) (-0.3044, -86.7019) (-0.0771, -87.2969) knots -0.994293 -0.994293 -0.994293 -0.994293 -0.994293 -0.994293 -0.9 -0.8 -0.7 -0.6 -0.5 -0.4 -0.3 -0.2 -0.1 -0.006357 -0.006357 -0.006357 -0.006357 -0.006357 -0.006357
  line L5 (-0.0771, -87.2969) -> (-0.0479, -87.5)
  line L6 (-0.0479, -87.5) -> (-0.0284, -87.4251)
  line L7 (-0.0284, -87.4251) -> (0, -87.5)
  line L8 (0, -87.5) -> (0, -87.3173)
  spline S2 degree 5 poles (0, -87.3173) (0.1588, -86.7166) (0.4926, -85.5292) (1.0191, -83.8882) (1.7672, -82.0144) (2.7817, -80.2473) (3.8935, -79.1086) (5.0974, -78.6698) (6.3967, -78.9545) (7.787, -79.9297) (9.2424, -81.5208) (10.4625, -83.2413) (11.4037, -84.7603) (12.0376, -85.8627) (12.3473, -86.4193) knots -0.994293 -0.994293 -0.994293 -0.994293 -0.994293 -0.994293 -0.9 -0.8 -0.7 -0.6 -0.5 -0.4 -0.3 -0.2 -0.1 -0.006357 -0.006357 -0.006357 -0.006357 -0.006357 -0.006357
  line L9 (12.3473, -86.4193) -> (12.4051, -86.6162)
  line L10 (12.4051, -86.6162) -> (12.4138, -86.5392)
  line L11 (12.4138, -86.5392) -> (12.4525, -86.6094)
  line L12 (12.4525, -86.6094) -> (12.4265, -86.4285)
  spline S3 degree 5 poles (12.4265, -86.4285) (12.4982, -85.8113) (12.6597, -84.5885) (12.9472, -82.8893) (13.4211, -80.9282) (14.1738, -79.0346) (15.1122, -77.7493) (16.2414, -77.1436) (17.568, -77.2405) (19.0829, -78.0079) (20.75, -79.3757) (22.2025, -80.905) (23.3503, -82.2746) (24.1346, -83.2756) (24.5204, -83.7825) knots -0.994293 -0.994293 -0.994293 -0.994293 -0.994293 -0.994293 -0.9 -0.8 -0.7 -0.6 -0.5 -0.4 -0.3 -0.2 -0.1 -0.006357 -0.006357 -0.006357 -0.006357 -0.006357 -0.006357
  line L13 (24.5204, -83.7825) -> (24.6056, -83.9691)
  line L14 (24.6056, -83.9691) -> (24.6033, -83.8917)
  line L15 (24.6033, -83.8917) -> (24.6516, -83.9556)
  line L16 (24.6516, -83.9556) -> (24.6001, -83.7803)
  spline S4 degree 5 poles (24.6001, -83.7803) (24.5832, -83.1592) (24.569, -81.9259) (24.6118, -80.203) (24.8018, -78.1944) (25.2773, -76.213) (26.0232, -74.8073) (27.0548, -74.047) (28.3817, -73.9542) (29.9904, -74.4981) (31.8351, -75.6147) (33.4905, -76.9218) (34.8215, -78.1141) (35.7403, -78.9933) (36.1943, -79.4401) knots -0.994293 -0.994293 -0.994293 -0.994293 -0.994293 -0.994293 -0.9 -0.8 -0.7 -0.6 -0.5 -0.4 -0.3 -0.2 -0.1 -0.006357 -0.006357 -0.006357 -0.006357 -0.006357 -0.006357
  line L17 (36.1943, -79.4401) -> (36.3052, -79.6127)
  line L18 (36.3052, -79.6127) -> (36.2919, -79.5364)
  line L19 (36.2919, -79.5364) -> (36.3488, -79.5928)
  line L20 (36.3488, -79.5928) -> (36.2729, -79.4266)
  spline S5 degree 5 poles (36.2729, -79.4266) (36.1678, -78.8142) (35.9782, -77.5954) (35.7754, -75.884) (35.6775, -73.8688) (35.8663, -71.8399) (36.4045, -70.3423) (37.3174, -69.443) (38.6176, -69.1623) (40.2873, -69.4718) (42.2722, -70.3145) (44.0967, -71.3726) (45.5838, -72.3634) (46.6185, -73.1028) (47.1314, -73.4805) knots -0.994293 -0.994293 -0.994293 -0.994293 -0.994293 -0.994293 -0.9 -0.8 -0.7 -0.6 -0.5 -0.4 -0.3 -0.2 -0.1 -0.006357 -0.006357 -0.006357 -0.006357 -0.006357 -0.006357
  line L21 (47.1314, -73.4805) -> (47.2657, -73.6356)
  line L22 (47.2657, -73.6356) -> (47.2417, -73.562)
  line L23 (47.2417, -73.562) -> (47.3061, -73.6097)
  line L24 (47.3061, -73.6097) -> (47.2073, -73.456)
  spline S6 degree 5 poles (47.2073, -73.456) (47.0161, -72.8648) (46.655, -71.6854) (46.2107, -70.0203) (45.827, -68.0395) (45.7251, -66.0044) (46.0448, -64.4455) (46.8203, -63.4254) (48.0673, -62.9624) (49.7641, -63.0312) (51.8487, -63.5828) (53.8052, -64.3705) (55.4182, -65.1396) (56.5476, -65.7243) (57.109, -66.0251) knots -0.994293 -0.994293 -0.994293 -0.994293 -0.994293 -0.994293 -0.9 -0.8 -0.7 -0.6 -0.5 -0.4 -0.3 -0.2 -0.1 -0.006357 -0.006357 -0.006357 -0.006357 -0.006357 -0.006357
  line L25 (57.109, -66.0251) -> (57.2641, -66.1595)
  line L26 (57.2641, -66.1595) -> (57.2298, -66.09)
  line L27 (57.2298, -66.09) -> (57.3003, -66.1281)
  line L28 (57.3003, -66.1281) -> (57.1807, -65.99)
  spline S7 degree 5 poles (57.1807, -65.99) (56.9073, -65.432) (56.382, -64.316) (55.7052, -62.7311) (55.0436, -60.8251) (54.6531, -58.8252) (54.7476, -57.2366) (55.3701, -56.1166) (56.5386, -55.4809) (58.2279, -55.3074) (60.3697, -55.5568) (62.4185, -56.0581) (64.1245, -56.5897) (65.3255, -57.0077) (65.9241, -57.2256) knots -0.994293 -0.994293 -0.994293 -0.994293 -0.994293 -0.994293 -0.9 -0.8 -0.7 -0.6 -0.5 -0.4 -0.3 -0.2 -0.1 -0.006357 -0.006357 -0.006357 -0.006357 -0.006357 -0.006357
  line L29 (65.9241, -57.2256) -> (66.0967, -57.3365)
  line L30 (66.0967, -57.3365) -> (66.0529, -57.2727)
  line L31 (66.0529, -57.2727) -> (66.1281, -57.3003)
  line L32 (66.1281, -57.3003) -> (65.99, -57.1807)
  spline S8 degree 5 poles (65.99, -57.1807) (65.64, -56.6673) (64.9613, -55.6374) (64.0658, -54.1649) (63.1396, -52.3725) (62.4685, -50.4485) (62.336, -48.8627) (62.7928, -47.6654) (63.8588, -46.8699) (65.5062, -46.4578) (67.6618, -46.3998) (69.761, -46.6044) (71.5254, -46.8878) (72.7737, -47.1307) (73.3971, -47.2612) knots -0.994293 -0.994293 -0.994293 -0.994293 -0.994293 -0.994293 -0.9 -0.8 -0.7 -0.6 -0.5 -0.4 -0.3 -0.2 -0.1 -0.006357 -0.006357 -0.006357 -0.006357 -0.006357 -0.006357
  line L33 (73.3971, -47.2612) -> (73.5838, -47.3464)
  line L34 (73.5838, -47.3464) -> (73.5313, -47.2894)
  line L35 (73.5313, -47.2894) -> (73.6097, -47.3061)
  line L36 (73.6097, -47.3061) -> (73.456, -47.2073)
  spline S9 degree 5 poles (73.456, -47.2073) (73.0365, -46.7489) (72.2181, -45.8261) (71.1222, -44.4961) (69.9504, -42.8537) (69.0122, -41.0448) (68.6554, -39.494) (68.9371, -38.2439) (69.8791, -37.3048) (71.4511, -36.6624) (73.5765, -36.2983) (75.6835, -36.202) (77.4702, -36.2315) (78.7403, -36.2942) (79.376, -36.3346) knots -0.994293 -0.994293 -0.994293 -0.994293 -0.994293 -0.994293 -0.9 -0.8 -0.7 -0.6 -0.5 -0.4 -0.3 -0.2 -0.1 -0.006357 -0.006357 -0.006357 -0.006357 -0.006357 -0.006357
  line L37 (79.376, -36.3346) -> (79.5729, -36.3924)
  line L38 (79.5729, -36.3924) -> (79.5128, -36.3435)
  line L39 (79.5128, -36.3435) -> (79.5928, -36.3488)
  line L40 (79.5928, -36.3488) -> (79.4266, -36.2729)
  spline S10 degree 5 poles (79.4266, -36.2729) (78.9461, -35.8789) (78.0047, -35.082) (76.7307, -33.9214) (75.3371, -32.4625) (74.151, -30.8056) (73.5772, -29.3213) (73.6781, -28.0438) (74.4769, -26.9802) (75.9415, -26.1207) (77.9934, -25.4578) (80.0652, -25.0626) (81.8379, -24.8375) (83.1041, -24.7188) (83.7391, -24.6684) knots -0.994293 -0.994293 -0.994293 -0.994293 -0.994293 -0.994293 -0.9 -0.8 -0.7 -0.6 -0.5 -0.4 -0.3 -0.2 -0.1 -0.006357 -0.006357 -0.006357 -0.006357 -0.006357 -0.006357
  line L41 (83.7391, -24.6684) -> (83.9421, -24.6976)
  line L42 (83.9421, -24.6976) -> (83.8757, -24.6577)
  line L43 (83.8757, -24.6577) -> (83.9556, -24.6516)
  line L44 (83.9556, -24.6516) -> (83.7803, -24.6001)
  spline S11 degree 5 poles (83.7803, -24.6001) (83.2487, -24.2785) (82.2035, -23.6237) (80.7772, -22.6562) (79.1902, -21.4105) (77.7804, -19.9392) (77.0011, -18.5517) (76.9192, -17.2729) (77.5585, -16.1064) (78.8858, -15.0472) (80.8225, -14.099) (82.817, -13.4131) (84.5397, -12.938) (85.776, -12.6403) (86.3974, -12.5) knots -0.994293 -0.994293 -0.994293 -0.994293 -0.994293 -0.994293 -0.9 -0.8 -0.7 -0.6 -0.5 -0.4 -0.3 -0.2 -0.1 -0.006357 -0.006357 -0.006357 -0.006357 -0.006357 -0.006357
  line L45 (86.3974, -12.5) -> (86.6025, -12.5)
  line L46 (86.6025, -12.5) -> (86.5312, -12.47)
  line L47 (86.5312, -12.47) -> (86.6094, -12.4525)
  line L48 (86.6094, -12.4525) -> (86.4285, -12.4265)
  spline S12 degree 5 poles (86.4285, -12.4265) (85.8565, -12.1839) (84.7287, -11.6844) (83.1793, -10.9298) (81.4312, -9.9227) (79.8263, -8.667) (78.8575, -7.4045) (78.5945, -6.1503) (79.0612, -4.9048) (80.2243, -3.6674) (82.0064, -2.4533) (83.883, -1.4905) (85.5204, -0.775) (86.7019, -0.3044) (87.2969, -0.0771) knots -0.994293 -0.994293 -0.994293 -0.994293 -0.994293 -0.994293 -0.9 -0.8 -0.7 -0.6 -0.5 -0.4 -0.3 -0.2 -0.1 -0.006357 -0.006357 -0.006357 -0.006357 -0.006357 -0.006357
  line L49 (87.2969, -0.0771) -> (87.5, -0.0479)
  line L50 (87.5, -0.0479) -> (87.4251, -0.0284)
  line L51 (87.4251, -0.0284) -> (87.5, 0)
  line L52 (87.5, 0) -> (87.3173, 0)
  spline S13 degree 5 poles (87.3173, 0) (86.7166, 0.1588) (85.5292, 0.4926) (83.8882, 1.0191) (82.0144, 1.7672) (80.2473, 2.7817) (79.1086, 3.8935) (78.6698, 5.0974) (78.9545, 6.3967) (79.9297, 7.787) (81.5208, 9.2424) (83.2413, 10.4625) (84.7603, 11.4037) (85.8627, 12.0376) (86.4193, 12.3473) knots -0.994293 -0.994293 -0.994293 -0.994293 -0.994293 -0.994293 -0.9 -0.8 -0.7 -0.6 -0.5 -0.4 -0.3 -0.2 -0.1 -0.006357 -0.006357 -0.006357 -0.006357 -0.006357 -0.006357
  line L53 (86.4193, 12.3473) -> (86.6162, 12.4051)
  line L54 (86.6162, 12.4051) -> (86.5392, 12.4138)
  line L55 (86.5392, 12.4138) -> (86.6094, 12.4525)
  line L56 (86.6094, 12.4525) -> (86.4285, 12.4265)
  spline S14 degree 5 poles (86.4285, 12.4265) (85.8113, 12.4982) (84.5885, 12.6597) (82.8893, 12.9472) (80.9282, 13.4211) (79.0346, 14.1738) (77.7493, 15.1122) (77.1436, 16.2414) (77.2405, 17.568) (78.0079, 19.0829) (79.3757, 20.75) (80.905, 22.2025) (82.2746, 23.3503) (83.2756, 24.1346) (83.7825, 24.5204) knots -0.994293 -0.994293 -0.994293 -0.994293 -0.994293 -0.994293 -0.9 -0.8 -0.7 -0.6 -0.5 -0.4 -0.3 -0.2 -0.1 -0.006357 -0.006357 -0.006357 -0.006357 -0.006357 -0.006357
  line L57 (83.7825, 24.5204) -> (83.9691, 24.6056)
  line L58 (83.9691, 24.6056) -> (83.8917, 24.6033)
  line L59 (83.8917, 24.6033) -> (83.9556, 24.6516)
  line L60 (83.9556, 24.6516) -> (83.7803, 24.6001)
  spline S15 degree 5 poles (83.7803, 24.6001) (83.1592, 24.5832) (81.9259, 24.569) (80.203, 24.6118) (78.1944, 24.8018) (76.213, 25.2773) (74.8073, 26.0232) (74.047, 27.0548) (73.9542, 28.3817) (74.4981, 29.9904) (75.6147, 31.8351) (76.9218, 33.4905) (78.1141, 34.8215) (78.9933, 35.7403) (79.4401, 36.1943) knots -0.994293 -0.994293 -0.994293 -0.994293 -0.994293 -0.994293 -0.9 -0.8 -0.7 -0.6 -0.5 -0.4 -0.3 -0.2 -0.1 -0.006357 -0.006357 -0.006357 -0.006357 -0.006357 -0.006357
  line L61 (79.4401, 36.1943) -> (79.6127, 36.3052)
  line L62 (79.6127, 36.3052) -> (79.5364, 36.2919)
  line L63 (79.5364, 36.2919) -> (79.5928, 36.3488)
  line L64 (79.5928, 36.3488) -> (79.4266, 36.2729)
  spline S16 degree 5 poles (79.4266, 36.2729) (78.8142, 36.1678) (77.5954, 35.9782) (75.884, 35.7754) (73.8688, 35.6775) (71.8399, 35.8663) (70.3423, 36.4045) (69.443, 37.3174) (69.1623, 38.6176) (69.4718, 40.2873) (70.3145, 42.2722) (71.3726, 44.0967) (72.3634, 45.5838) (73.1028, 46.6185) (73.4805, 47.1314) knots -0.994293 -0.994293 -0.994293 -0.994293 -0.994293 -0.994293 -0.9 -0.8 -0.7 -0.6 -0.5 -0.4 -0.3 -0.2 -0.1 -0.006357 -0.006357 -0.006357 -0.006357 -0.006357 -0.006357
  line L65 (73.4805, 47.1314) -> (73.6356, 47.2657)
  line L66 (73.6356, 47.2657) -> (73.562, 47.2417)
  line L67 (73.562, 47.2417) -> (73.6097, 47.3061)
  line L68 (73.6097, 47.3061) -> (73.456, 47.2073)
  spline S17 degree 5 poles (73.456, 47.2073) (72.8648, 47.0161) (71.6854, 46.655) (70.0203, 46.2107) (68.0395, 45.827) (66.0044, 45.7251) (64.4455, 46.0448) (63.4254, 46.8203) (62.9624, 48.0673) (63.0312, 49.7641) (63.5828, 51.8487) (64.3705, 53.8052) (65.1396, 55.4182) (65.7243, 56.5476) (66.0251, 57.109) knots -0.994293 -0.994293 -0.994293 -0.994293 -0.994293 -0.994293 -0.9 -0.8 -0.7 -0.6 -0.5 -0.4 -0.3 -0.2 -0.1 -0.006357 -0.006357 -0.006357 -0.006357 -0.006357 -0.006357
  line L69 (66.0251, 57.109) -> (66.1595, 57.2641)
  line L70 (66.1595, 57.2641) -> (66.09, 57.2298)
  line L71 (66.09, 57.2298) -> (66.1281, 57.3003)
  line L72 (66.1281, 57.3003) -> (65.99, 57.1807)
  spline S18 degree 5 poles (65.99, 57.1807) (65.432, 56.9073) (64.316, 56.382) (62.7311, 55.7052) (60.8251, 55.0436) (58.8252, 54.6531) (57.2366, 54.7476) (56.1166, 55.3701) (55.4809, 56.5386) (55.3074, 58.2279) (55.5568, 60.3697) (56.0581, 62.4185) (56.5897, 64.1245) (57.0077, 65.3255) (57.2256, 65.9241) knots -0.994293 -0.994293 -0.994293 -0.994293 -0.994293 -0.994293 -0.9 -0.8 -0.7 -0.6 -0.5 -0.4 -0.3 -0.2 -0.1 -0.006357 -0.006357 -0.006357 -0.006357 -0.006357 -0.006357
  line L73 (57.2256, 65.9241) -> (57.3365, 66.0967)
  line L74 (57.3365, 66.0967) -> (57.2727, 66.0529)
  line L75 (57.2727, 66.0529) -> (57.3003, 66.1281)
  line L76 (57.3003, 66.1281) -> (57.1807, 65.99)
  spline S19 degree 5 poles (57.1807, 65.99) (56.6673, 65.64) (55.6374, 64.9613) (54.1649, 64.0658) (52.3725, 63.1396) (50.4485, 62.4685) (48.8627, 62.336) (47.6654, 62.7928) (46.8699, 63.8588) (46.4578, 65.5062) (46.3998, 67.6618) (46.6044, 69.761) (46.8878, 71.5254) (47.1307, 72.7737) (47.2612, 73.3971) knots -0.994293 -0.994293 -0.994293 -0.994293 -0.994293 -0.994293 -0.9 -0.8 -0.7 -0.6 -0.5 -0.4 -0.3 -0.2 -0.1 -0.006357 -0.006357 -0.006357 -0.006357 -0.006357 -0.006357
  line L77 (47.2612, 73.3971) -> (47.3464, 73.5838)
  line L78 (47.3464, 73.5838) -> (47.2894, 73.5313)
  line L79 (47.2894, 73.5313) -> (47.3061, 73.6097)
  line L80 (47.3061, 73.6097) -> (47.2073, 73.456)
  spline S20 degree 5 poles (47.2073, 73.456) (46.7489, 73.0365) (45.8261, 72.2181) (44.4961, 71.1222) (42.8537, 69.9504) (41.0448, 69.0122) (39.494, 68.6554) (38.2439, 68.9371) (37.3048, 69.8791) (36.6624, 71.4511) (36.2983, 73.5765) (36.202, 75.6835) (36.2315, 77.4702) (36.2942, 78.7403) (36.3346, 79.376) knots -0.994293 -0.994293 -0.994293 -0.994293 -0.994293 -0.994293 -0.9 -0.8 -0.7 -0.6 -0.5 -0.4 -0.3 -0.2 -0.1 -0.006357 -0.006357 -0.006357 -0.006357 -0.006357 -0.006357
  line L81 (36.3346, 79.376) -> (36.3924, 79.5729)
  line L82 (36.3924, 79.5729) -> (36.3435, 79.5128)
  line L83 (36.3435, 79.5128) -> (36.3488, 79.5928)
  line L84 (36.3488, 79.5928) -> (36.2729, 79.4266)
  spline S21 degree 5 poles (36.2729, 79.4266) (35.8789, 78.9461) (35.082, 78.0047) (33.9214, 76.7307) (32.4625, 75.3371) (30.8056, 74.151) (29.3213, 73.5772) (28.0438, 73.6781) (26.9802, 74.4769) (26.1207, 75.9415) (25.4578, 77.9934) (25.0626, 80.0652) (24.8375, 81.8379) (24.7188, 83.1041) (24.6684, 83.7391) knots -0.994293 -0.994293 -0.994293 -0.994293 -0.994293 -0.994293 -0.9 -0.8 -0.7 -0.6 -0.5 -0.4 -0.3 -0.2 -0.1 -0.006357 -0.006357 -0.006357 -0.006357 -0.006357 -0.006357
  line L85 (24.6684, 83.7391) -> (24.6976, 83.9421)
  line L86 (24.6976, 83.9421) -> (24.6577, 83.8757)
  line L87 (24.6577, 83.8757) -> (24.6516, 83.9556)
  line L88 (24.6516, 83.9556) -> (24.6001, 83.7803)
  spline S22 degree 5 poles (24.6001, 83.7803) (24.2785, 83.2487) (23.6237, 82.2035) (22.6562, 80.7772) (21.4105, 79.1902) (19.9392, 77.7804) (18.5517, 77.0011) (17.2729, 76.9192) (16.1064, 77.5585) (15.0472, 78.8858) (14.099, 80.8225) (13.4131, 82.817) (12.938, 84.5397) (12.6403, 85.776) (12.5, 86.3974) knots -0.994293 -0.994293 -0.994293 -0.994293 -0.994293 -0.994293 -0.9 -0.8 -0.7 -0.6 -0.5 -0.4 -0.3 -0.2 -0.1 -0.006357 -0.006357 -0.006357 -0.006357 -0.006357 -0.006357
  line L89 (12.5, 86.3974) -> (12.5, 86.6025)
  line L90 (12.5, 86.6025) -> (12.47, 86.5312)
  line L91 (12.47, 86.5312) -> (12.4525, 86.6094)
  line L92 (12.4525, 86.6094) -> (12.4265, 86.4285)
  spline S23 degree 5 poles (12.4265, 86.4285) (12.1839, 85.8565) (11.6844, 84.7287) (10.9298, 83.1793) (9.9227, 81.4312) (8.667, 79.8263) (7.4045, 78.8575) (6.1503, 78.5945) (4.9048, 79.0612) (3.6674, 80.2243) (2.4533, 82.0064) (1.4905, 83.883) (0.775, 85.5204) (0.3044, 86.7019) (0.0771, 87.2969) knots -0.994293 -0.994293 -0.994293 -0.994293 -0.994293 -0.994293 -0.9 -0.8 -0.7 -0.6 -0.5 -0.4 -0.3 -0.2 -0.1 -0.006357 -0.006357 -0.006357 -0.006357 -0.006357 -0.006357
  line L93 (0.0771, 87.2969) -> (0.0479, 87.5)
  line L94 (0.0479, 87.5) -> (0.0284, 87.4251)
  line L95 (0.0284, 87.4251) -> (0, 87.5)
  line L96 (0, 87.5) -> (0, 87.3173)
  spline S24 degree 5 poles (0, 87.3173) (-0.1588, 86.7166) (-0.4926, 85.5292) (-1.0191, 83.8882) (-1.7672, 82.0144) (-2.7817, 80.2473) (-3.8935, 79.1086) (-5.0974, 78.6698) (-6.3967, 78.9545) (-7.787, 79.9297) (-9.2424, 81.5208) (-10.4625, 83.2413) (-11.4037, 84.7603) (-12.0376, 85.8627) (-12.3473, 86.4193) knots -0.994293 -0.994293 -0.994293 -0.994293 -0.994293 -0.994293 -0.9 -0.8 -0.7 -0.6 -0.5 -0.4 -0.3 -0.2 -0.1 -0.006357 -0.006357 -0.006357 -0.006357 -0.006357 -0.006357
  line L97 (-12.3473, 86.4193) -> (-12.4051, 86.6162)
  line L98 (-12.4051, 86.6162) -> (-12.4138, 86.5392)
  line L99 (-12.4138, 86.5392) -> (-12.4525, 86.6094)
  line L100 (-12.4525, 86.6094) -> (-12.4265, 86.4285)
  spline S25 degree 5 poles (-12.4265, 86.4285) (-12.4982, 85.8113) (-12.6597, 84.5885) (-12.9472, 82.8893) (-13.4211, 80.9282) (-14.1738, 79.0346) (-15.1122, 77.7493) (-16.2414, 77.1436) (-17.568, 77.2405) (-19.0829, 78.0079) (-20.75, 79.3757) (-22.2025, 80.905) (-23.3503, 82.2746) (-24.1346, 83.2756) (-24.5204, 83.7825) knots -0.994293 -0.994293 -0.994293 -0.994293 -0.994293 -0.994293 -0.9 -0.8 -0.7 -0.6 -0.5 -0.4 -0.3 -0.2 -0.1 -0.006357 -0.006357 -0.006357 -0.006357 -0.006357 -0.006357
  line L101 (-24.5204, 83.7825) -> (-24.6056, 83.9691)
  line L102 (-24.6056, 83.9691) -> (-24.6033, 83.8917)
  line L103 (-24.6033, 83.8917) -> (-24.6516, 83.9556)
  line L104 (-24.6516, 83.9556) -> (-24.6001, 83.7803)
  spline S26 degree 5 poles (-24.6001, 83.7803) (-24.5832, 83.1592) (-24.569, 81.9259) (-24.6118, 80.203) (-24.8018, 78.1944) (-25.2773, 76.213) (-26.0232, 74.8073) (-27.0548, 74.047) (-28.3817, 73.9542) (-29.9904, 74.4981) (-31.8351, 75.6147) (-33.4905, 76.9218) (-34.8215, 78.1141) (-35.7403, 78.9933) (-36.1943, 79.4401) knots -0.994293 -0.994293 -0.994293 -0.994293 -0.994293 -0.994293 -0.9 -0.8 -0.7 -0.6 -0.5 -0.4 -0.3 -0.2 -0.1 -0.006357 -0.006357 -0.006357 -0.006357 -0.006357 -0.006357
  line L105 (-36.1943, 79.4401) -> (-36.3052, 79.6127)
  line L106 (-36.3052, 79.6127) -> (-36.2919, 79.5364)
  line L107 (-36.2919, 79.5364) -> (-36.3488, 79.5928)
  line L108 (-36.3488, 79.5928) -> (-36.2729, 79.4266)
  spline S27 degree 5 poles (-36.2729, 79.4266) (-36.1678, 78.8142) (-35.9782, 77.5954) (-35.7754, 75.884) (-35.6775, 73.8688) (-35.8663, 71.8399) (-36.4045, 70.3423) (-37.3174, 69.443) (-38.6176, 69.1623) (-40.2873, 69.4718) (-42.2722, 70.3145) (-44.0967, 71.3726) (-45.5838, 72.3634) (-46.6185, 73.1028) (-47.1314, 73.4805) knots -0.994293 -0.994293 -0.994293 -0.994293 -0.994293 -0.994293 -0.9 -0.8 -0.7 -0.6 -0.5 -0.4 -0.3 -0.2 -0.1 -0.006357 -0.006357 -0.006357 -0.006357 -0.006357 -0.006357
  line L109 (-47.1314, 73.4805) -> (-47.2657, 73.6356)
  line L110 (-47.2657, 73.6356) -> (-47.2417, 73.562)